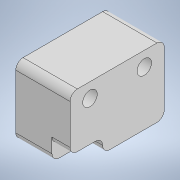
# Autodesk Inventor part: 29_Lasercable_holder_A
Saved by Autodesk Inventor 2022 (Build 260153000, 153)
## iProperties
Created: 2023-01-15
Part Number: 29_Lasercable_holder_A
Material: Generic
Document SubType Name: Modeling
Designer: Max
Density: 1 g/cm^3
Appearance: Default
Author: Max
Autodesk Inventor part; units mm, degrees
ref_plane "YZ Plane" through (0, 0, 0) normal (1, 0, 0) x (0, 1, 0)
ref_plane "XZ Plane" through (0, 0, 0) normal (0, 1, 0) x (-1, 0, 0)
ref_plane "XY Plane" through (0, 0, 0) normal (0, 0, 1) x (1, 0, 0)
sketch "Sketch1" plane through (0, 0, 0) normal (0, 1, 0) x (-1, 0, 0)
  line L0 (-7.5, 13) -> (7.5, 13)
  line L1 (7.5, 13) -> (7.5, -13)
  line L2 (7.5, -13) -> (-7.5, -13)
  line L3 (-7.5, -13) -> (-7.5, 13)
  line L4 (-7.5, 13) -> (7.5, -13) construction
  line L5 (7.5, 13) -> (-7.5, -13) construction
  point P0 (0, 0)
  dimension "d0" = 15
  dimension "d1" = 26
  constraints: 12 end point, 2 midpoint, 2 parallel, 1 horizontal, 1 perpendicular
  measures "d0" distance of L1.end L2.end
  measures "d1" distance of L0.end L1.end
extrude "Extrusion1" add sketch "Sketch1" along normal blind 19
sketch "Sketch2" plane through (7.5, 0, 13) normal (1, 0, 0) x (0, 0, -1)
  line L0 (13, -3.8) -> (13, 22.8) projected
  circle A0 centre (5.5, 15) radius 2
  circle A1 centre (20.5, 15) radius 2
  line L1 (0, 0) -> (26, 0) projected
  point P0 (13, 0)
  dimension "d4" = 15
  dimension "d5" = 15
  constraints: 2 centre point, 1 equal radius, 1 other
  measures "d4" distance of A1.centre A0.centre
  measures "d5" distance from line of A0.centre L1
extrude "Extrusion2" cut sketch "Sketch2" against normal through all
sketch "Sketch3" plane through (7.5, 0, 13) normal (1, 0, 0) x (0, 0, -1)
  line L0 (26, 0) -> (0, 0) projected
  line L1 (0, 0) -> (9, 0)
  line L2 (9, 0) -> (9, 4)
  line L3 (9, 4) -> (0, 4)
  line L4 (0, 4) -> (0, 0)
  point P0 (13, 0)
  dimension "d8" = 4
  dimension "d9" = 9
  constraints: 8 end point, 2 parallel, 1 horizontal, 1 perpendicular
  measures "d8" distance of L2.end L1.end
  measures "d9" distance between parallel lines of L4 L2
extrude "Extrusion3" cut sketch "Sketch3" against normal blind 5
fillet "Fillet1" radius 2 7 edges at (0, 19, -13) (0, 19, 13) (0, 0, -13) (-2.5, 0, 13) (5, 4, 13) (5, 4, 4) (5, 0, 4)
body "Solid1"
